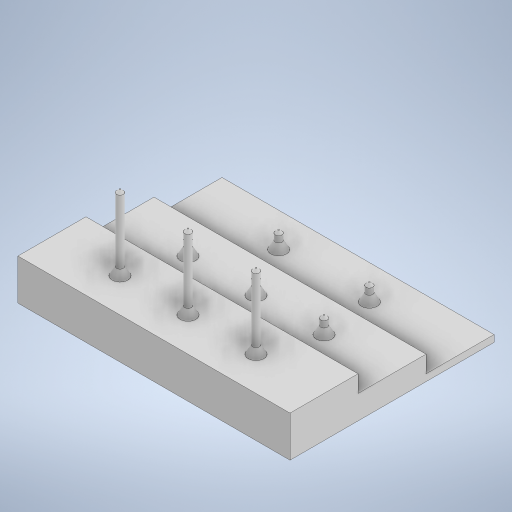
# Autodesk Inventor part: Part1
Saved by Autodesk Inventor 2024 (Build 280153000, 153)
## iProperties
Created: 2024-02-22
Part Number: Part1
Material: Generic
Document SubType Name: Modeling
Designer: evmgm
Density: 1 g/cm^3
Appearance: Default
Author: evmgm
Autodesk Inventor part; units mm, degrees
ref_plane "YZ Plane" through (0, 0, 0) normal (1, 0, 0) x (0, 1, 0)
ref_plane "XZ Plane" through (0, 0, 0) normal (0, 1, 0) x (-1, 0, 0)
ref_plane "XY Plane" through (0, 0, 0) normal (0, 0, 1) x (1, 0, 0)
sketch "Sketch1" plane through (0, 0, 0) normal (0, 1, 0) x (-1, 0, 0)
  line L0 (0, 0) -> (-400, 0)
  line L1 (-400, 0) -> (-400, -300)
  line L2 (-400, -300) -> (0, -300)
  line L3 (0, -300) -> (0, 0)
  line L4 (0, -200) -> (-400, -200)
  line L5 (0, -100) -> (-400, -100)
  dimension "d0" = 400
  dimension "d1" = 300
  dimension "d21" = 100
  dimension "d22" = 100
  constraints: 12 end point, 4 point on line, 3 parallel, 2 perpendicular, 1 horizontal
  measures "d0" distance of L2.end L1.end
  measures "d1" distance of L1.end L0.end
  measures "d21" distance between parallel lines of L2 L4
  measures "d22" distance between parallel lines of L4 L5
extrude "Extrusion1" add sketch "Sketch1" along normal blind 10 contours L3 L2 L1 L4
extrude "Extrusion2" add sketch "Sketch1" along normal blind 35 contours L3 L4 L1 L5
extrude "Extrusion3" add sketch "Sketch1" along normal blind 60 contours L3 L5 L1 L0
sketch "Sketch2" plane through (0, 60, 0) normal (0, 1, 0) x (1, 0, 0)
  line L0 (0, 300) -> (0, 0) projected
  line L1 (0, 50) -> (400, 50) construction
  line L2 (400, 0) -> (400, 300) projected
  line L3 (0, 0) -> (400, 0) projected
  line L4 (0, 100) -> (0, 0) projected
  circle A0 centre (100, 50) radius 5
  circle A1 centre (200, 50) radius 5
  circle A2 centre (300, 50) radius 5
  point P0 (0, 50)
  dimension "d30" = 50
  dimension "d32" = 100
  dimension "d33" = 100
  dimension "d34" = 100
  dimension "d35" = 10
  dimension "d36" = 10
  dimension "d37" = 10
  constraints: 4 point on line, 3 centre point, 3 coincident, 2 end point, 2 midpoint, 1 horizontal
  measures "d30" distance between parallel lines of L3 L1
  measures "d32" distance of point (0, 50) point (100, 50)
  measures "d33" distance of point (200, 50) point (100, 50)
  measures "d34" distance of point (200, 50) point (300, 50)
  measures "d35" diameter of A0
  measures "d36" diameter of A1
  measures "d37" diameter of A2
extrude "Extrusion4" add sketch "Sketch2" along normal blind 110
chamfer "Chamfer1" distance 4 angle 45 3 edges at (295, 170, -50) (195, 170, -50) (95, 170, -50)
sketch "Sketch3" plane through (0, 35, 0) normal (0, 1, 0) x (1, 0, 0)
  line L0 (0, 200) -> (0, 100) projected
  line L1 (0, 150) -> (400, 150) construction
  line L2 (400, 0) -> (400, 300) projected
  circle A0 centre (100, 150) radius 5
  circle A1 centre (200, 150) radius 5
  circle A2 centre (300, 150) radius 5
  point P0 (0, 0)
  dimension "d43" = 100
  dimension "d44" = 100
  dimension "d45" = 100
  dimension "d46" = 10
  dimension "d47" = 10
  dimension "d48" = 10
  constraints: 4 midpoint, 3 centre point, 3 coincident, 2 end point, 2 point on line
  measures "d43" distance of point (0, 150) point (100, 150)
  measures "d44" distance of point (300, 150) point (200, 150)
  measures "d45" distance of point (200, 150) point (100, 150)
  measures "d46" diameter of A0
  measures "d47" diameter of A1
  measures "d48" diameter of A2
extrude "Extrusion5" add sketch "Sketch3" along normal blind 25
sketch "Sketch4" plane through (0, 10, 0) normal (0, 1, 0) x (1, 0, 0)
  line L0 (0, 300) -> (0, 200) projected
  line L1 (0, 250) -> (400, 250) construction
  line L2 (400, 0) -> (400, 300) projected
  circle A0 centre (133.3333, 250) radius 5
  circle A1 centre (266.6667, 250) radius 5
  point P0 (0, 0)
  dimension "d51" = 133.3333
  dimension "d52" = 133.3333
  dimension "d53" = 10
  dimension "d54" = 10
  constraints: 3 point on line, 2 centre point, 2 coincident, 2 end point, 2 midpoint, 1 horizontal
  measures "d51" distance of point (0, 250) point (133.333, 250)
  measures "d52" distance of point (266.667, 250) point (133.333, 250)
  measures "d53" diameter of A0
  measures "d54" diameter of A1
extrude "Extrusion6" add sketch "Sketch4" along normal blind 25
chamfer "Chamfer2" distance 4 angle 45 5 edges at (295, 60, -150) (261.6667, 35, -250) (128.3333, 35, -250) (95, 60, -150) (195, 60, -150)
chamfer "Chamfer3" distance 6.5 angle 61.2 1 edges at (295, 60, -50) measured on face at (200.2009, 60, -84.9878)
chamfer "Chamfer4" distance 6.5 angle 61.2 2 edges at (195, 60, -50) (95, 60, -50) measured on face at (200.2009, 60, -84.9878)
chamfer "Chamfer5" distance 6.5 angle 61.2 3 edges at (295, 35, -150) (195, 35, -150) (95, 35, -150) measured on face at (200.2009, 35, -184.9878)
chamfer "Chamfer6" distance 6.5 angle 61.2 2 edges at (128.3333, 10, -250) (261.6667, 10, -250) measured on face at (222.0213, 10, -215.0122)
body "Solid1"
